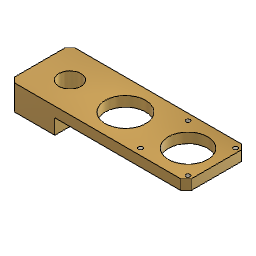
BC linear drive v5 (Autodesk Fusion 360 archive; units mm, degrees)
design "BC linear drive plate"
Autodesk Fusion 360 part; units mm, degrees
note: some values were not read from the file. Set by a fixed rule: the direction of a hole.
sketch "Sketch1" plane through (0, 0, 0) normal (0, 1, 0) x (1, 0, 0)
  circle A0 centre (0, 0) radius 20
  circle A1 centre (-55, 0) radius 16 construction
  circle A2 centre (-55, 0) radius 11
  line L0 (0, 0) -> (-55, 0) construction
  line L1 (-85, 30) -> (90, 30)
  line L2 (90, 30) -> (90, -30)
  line L3 (90, -30) -> (-85, -30)
  line L4 (-85, -30) -> (-85, 30)
  line L5 (-40, 30) -> (-40, -30)
  line L6 (-66.3137, -11.3137) -> (-43.6863, 11.3137) construction
  line L7 (-66.3137, 11.3137) -> (-43.6863, -11.3137) construction
  line L8 (-55, 16) -> (-55, -16) construction
  line L9 (38.43, -23.57) -> (85.57, -23.57) construction
  line L10 (85.57, -23.57) -> (85.57, 23.57) construction
  line L11 (85.57, 23.57) -> (38.43, 23.57) construction
  line L12 (38.43, 23.57) -> (38.43, -23.57) construction
  line L13 (38.43, 23.57) -> (85.57, -23.57) construction
  circle A3 centre (62, 0) radius 19.5
  point P0 (-66.3137, 11.3137)
  point P1 (-55, 16)
  point P2 (-43.6863, 11.3137)
  point P3 (-43.6863, -11.3137)
  point P4 (-55, -16)
  point P5 (-66.3137, -11.3137)
  dimension "d1" = 32
  dimension "d2" = 22
  dimension "d3" = 55
  dimension "d4" = 40
  dimension "d5" = 60
  dimension "d6" = 30
  dimension "d7" = 90
  dimension "d8" = 15
  dimension "d9" = 45
  dimension "d20" = 47.14
  dimension "d22" = 39
  dimension "d27" = 62
  constraint coincident A0.centre L0.start
  constraint concentric A1 A2
  constraint coincident A1.centre A2.centre
  constraint horizontal L0
  constraint horizontal L1
  constraint vertical L2
  constraint horizontal L3
  constraint vertical L4
  constraint symmetric L0 L1 L3
  constraint coincident L1 L5.start
  constraint coincident L3 L5.end
  constraint perpendicular L3 L5
  constraint coincident A1 P5
  constraint coincident A1 P2
  constraint coincident A1 P0
  constraint coincident A1 P3
  constraint coincident A1 P1
  constraint coincident A1 P4
  constraint coincident A1.centre L6
  constraint perpendicular L6 L7
  constraint coincident A1.centre L7
  constraint vertical L8
  constraint coincident A1.centre L8
  constraint coincident P0 L7.start
  constraint coincident P1 L8.start
  constraint coincident P2 L6.end
  constraint coincident P3 L7.end
  constraint coincident P4 L8.end
  constraint coincident P5 L6.start
  constraint horizontal L9
  constraint vertical L10
  constraint horizontal L11
  constraint vertical L12
  constraint equal L9 L12
  constraint symmetric L0 L9 L11
  constraint midpoint L13 A3.centre
  measures "d1" diameter of A1
  measures "d2" diameter of A2
  measures "d3" distance of A0.centre A1.centre
  measures "d4" diameter of A0
  measures "d5" distance of L1.start L3.end
  measures "d6" distance of A1.centre L4
  measures "d7" distance of A0.centre L2
  measures "d8" distance of A1.centre L5
  measures "d9" angle of L7 L8
  measures "d20" distance of L9.start L9.end
  measures "d22" diameter of A3
  measures "d27" distance of A0.centre A3.centre
extrude "Extrude1" add sketch "Sketch1" along normal blind 25
extrude "Extrude3" cut sketch "Sketch1" along normal blind 15 contours L1 L2 L3 L5 | A3
hole "Hole1" at (-66.3137, 0, 11.3137) at (-55, 0, 16) at (-66.3137, 0, -11.3137) at (-55, 0, -16) at (-43.6863, 0, -11.3137) at (-43.6863, 0, 11.3137) direction (0, 1, 0) diameter 3.332 depth 15 tip angle 118
thread "Thread1" "ISO Metric profile 4.0 M4x0.7 6H"
hole "Hole2" at (38.43, 0, 23.57) at (38.43, 0, -23.57) at (85.57, 0, 23.57) at (85.57, 0, -23.57) direction (0, 1, 0) diameter 4.234 depth 60 tip angle 118
thread "Thread2" "ISO Metric profile 5.0 M5x0.8 6H"
chamfer "Chamfer1" distance 5 angle 45 4 edges at (-85, 12.5, -30) (-85, 12.5, 30) (90, 20, -30) (90, 20, 30)

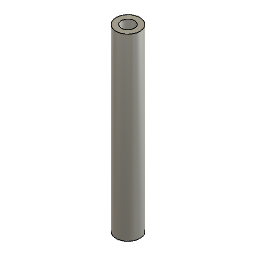
design "BC linaer drive motor spacer"
Autodesk Fusion 360 part; units mm, degrees
cylinder "CylinderPrimitive1" add diameter 10 height 75 placed x (1, 0, 0) y (0, 0, -1) z (0, 1, 0) at (0, 0, 0)
hole "Hole1" at (0, 0, 0) direction (0, 1, 0) diameter 5.5 end through all

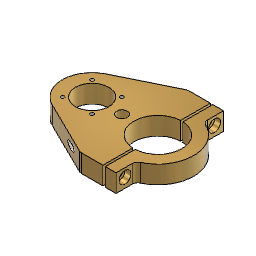
design "BC linear drive top bearing fixture"
Autodesk Fusion 360 part; units mm, degrees
sketch "Sketch1" plane through (0, 0, 0) normal (0, 1, 0) x (1, 0, 0)
  circle A0 centre (0, 0) radius 17.5 construction
  line L0 (-12.3744, 12.3744) -> (12.3744, 12.3744) construction
  line L1 (12.3744, 12.3744) -> (12.3744, -12.3744) construction
  line L2 (12.3744, -12.3744) -> (-12.3744, -12.3744) construction
  line L3 (-12.3744, -12.3744) -> (-12.3744, 12.3744) construction
  circle A1 centre (0, 0) radius 14
  circle A2 centre (55, 0) radius 20
  line L4 (65, 28.2843) -> (65, 45)
  line L5 (65, 45) -> (35, 45)
  line L6 (35, 45) -> (-11.0043, 22.4478)
  arc A3 (-11.0043, 22.4478) -> (-25, 0) centre (0, 0) ccw
  arc A4 (85, 0) -> (65, 28.2843) centre (55, 0) ccw
  line L7 (1.75, 0) -> (22.5, 0)
  arc A5 (65, -28.2843) -> (85, 0) centre (55, 0) ccw
  line L8 (65, -28.2843) -> (65, -45)
  line L9 (65, -45) -> (35, -45)
  line L10 (35, -45) -> (-11.0043, -22.4478)
  arc A6 (-25, 0) -> (-11.0043, -22.4478) centre (0, 0) ccw
  point P0 (25, 0)
  dimension "d1" = 35
  dimension "d2" = 28
  dimension "d3" = 40
  dimension "d4" = 55
  dimension "d5" = 25
  dimension "d6" = 30
  dimension "d7" = 10
  dimension "d8" = 30
  dimension "d9" = 45
  dimension "d31" = 30
  constraint coincident A0.centre A1.centre
  constraint horizontal L0
  constraint vertical L1
  constraint horizontal L2
  constraint vertical L3
  constraint coincident A0 L1.end
  constraint coincident A0 L0.start
  constraint equal L0 L1
  constraint coincident A0 L0.end
  constraint concentric A0 A1
  constraint horizontal A0.centre A2.centre
  constraint vertical L4
  constraint perpendicular L4 L5
  constraint tangent L6 A3
  constraint coincident A2.centre A4.centre
  constraint horizontal A2.centre A4.start
  constraint horizontal A0.centre A3.end
  constraint symmetric L4.start L7 A5.start
  constraint symmetric L4.end L7 L8.end
  constraint symmetric L5.end L7 L9.end
  constraint symmetric L6.end L7 L10.end
  constraint symmetric A3.end L7 A6.start
  constraint symmetric A3 L7 A6
  constraint symmetric A4.start L7 A5.end
  constraint symmetric A4 L7 A5
  constraint horizontal A2.centre P0
  measures "d1" diameter of A0
  measures "d2" diameter of A1
  measures "d3" diameter of A2
  measures "d4" distance of A0.centre A2.centre
  measures "d5" radius of A3
  measures "d6" radius of A4
  measures "d7" distance of A2.centre L4
  measures "d8" distance of L4.end L5.end
  measures "d9" distance of A2.centre L5
  measures "d31" distance of A2.centre P0
extrude "Extrude1" add sketch "Sketch1" along normal blind 15 makes body 1
hole "Hole1" at (-12.3744, 0, 12.3744) at (12.3744, 0, 12.3744) at (12.3744, 0, -12.3744) at (-12.3744, 0, -12.3744) direction (0, 1, 0) diameter 2.93 end through all bodies 1
thread "Thread2" "ISO Metric profile 3.5 M3.5x0.6 6H"
ref_plane "WorkPlane1" through (55, 0, 0) normal (1, 0, 0) x (0, 1, 0)
sketch "Sketch2" plane through (55, 0, 0) normal (1, 0, 0) x (0, 0, -1)
  line L0 (-52.531, 37.047) -> (45, 37.047)
  line L1 (45, 37.047) -> (45, -15)
  line L2 (45, -15) -> (-52.531, -15)
  line L3 (-52.531, -15) -> (-52.531, 37.047)
  constraint horizontal L0
  constraint vertical L1
  constraint horizontal L2
  constraint vertical L3
extrude "Extrude2" cut sketch "Sketch2" along normal mid plane 2 bodies 1 makes body 2 at (73.8112, 10, -23.3696)
sketch "Sketch3" plane through (65, 0, 0) normal (1, 0, 0) x (0, 0, -1)
  line L0 (28.2843, 0) -> (45, 0)
  line L1 (45, 0) -> (45, 15)
  line L2 (45, 15) -> (28.2843, 15)
  line L3 (28.2843, 15) -> (28.2843, 0)
  point P0 (37.5, 8)
  dimension "d23" = 7.5
  measures "d23" distance of L1 P0
hole "Hole2" at (65, 8, -37.5) direction (-1, 0, 0) diameter 5.5 depth 10 tip angle 180 counterbore diameter 10 counterbore depth 5 bodies 2
hole "Hole3" at (65, 8, -37.5) direction (-1, 0, 0) diameter 5.029 end through all bodies 1
thread "Thread1" "ISO Metric profile 5.5 M5.5x0.5 6H"
mirror "Mirror1" about plane through (0, 0, 0) normal (0, 0, 1) of "Hole2", "Hole3"
fillet "Fillet1" radius 5 4 edges at (35, 7.5, -45) (35, 7.5, 45) (65, 7.5, -28.2843) (65, 7.5, 28.2843) on bodies 1 2
hole "Hole4" at (25, 0, 0) direction (0, 1, 0) diameter 9 end through all bodies 1
copy_body "Body->Comp1" bodies 1 removing the originals makes body 3 in component "console"
copy_body "Body->Comp2" bodies 2 removing the originals makes body 4 in component "brace"
component "console" placed x (1, 0, 0) y (0, 1, 0) z (0, 0, 1) at (0, 0, 0)
component "brace" placed x (1, 0, 0) y (0, 1, 0) z (0, 0, 1) at (0, 0, 0)
named bodies: "console", "brace"

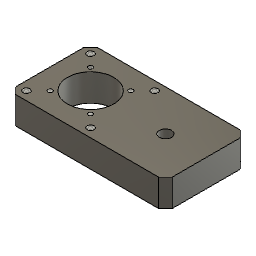
design "BC linear drive bottom bracket"
Autodesk Fusion 360 part; units mm, degrees
sketch "Sketch1" plane through (0, 0, 0) normal (0, 1, 0) x (1, 0, 0)
  circle A0 centre (-55, 0) radius 17
  line L0 (-78.57, 23.57) -> (-31.43, 23.57) construction
  line L1 (-31.43, 23.57) -> (-31.43, -23.57) construction
  line L2 (-31.43, -23.57) -> (-78.57, -23.57) construction
  line L3 (-78.57, -23.57) -> (-78.57, 23.57) construction
  line L4 (-78.57, -23.57) -> (-31.43, 23.57) construction
  line L5 (-85, 30) -> (30, 30)
  line L6 (30, 30) -> (30, -30)
  line L7 (30, -30) -> (-85, -30)
  line L8 (-85, -30) -> (-85, 30)
  line L9 (0, 0) -> (-55, 0) construction
  circle A1 centre (-55, 0) radius 21 construction
  line L10 (-78.57, 23.57) -> (-31.43, -23.57) construction
  line L11 (-55, 23.57) -> (-55, -23.57) construction
  line L12 (-78.57, 0) -> (-31.43, 0) construction
  point P0 (-55, 21)
  point P1 (-69.8492, 14.8492)
  point P2 (-76, 0)
  point P3 (-69.8492, -14.8492)
  point P4 (-55, -21)
  point P5 (-40.1508, -14.8492)
  point P6 (-40.1508, 14.8492)
  point P7 (-34, 0)
  dimension "d2" = 34
  dimension "d3" = 55
  dimension "d4" = 47.14
  dimension "d5" = 30
  dimension "d6" = 30
  dimension "d7" = 60
  dimension "d20" = 42
  constraint horizontal L0
  constraint vertical L1
  constraint horizontal L2
  constraint vertical L3
  constraint equal L2 L3
  constraint midpoint A0.centre L4
  constraint horizontal L5
  constraint vertical L6
  constraint horizontal L7
  constraint vertical L8
  constraint coincident L9.start origin
  constraint coincident A0.centre L9.end
  constraint symmetric L5 L7 L9
  constraint midpoint L0 L11.start
  constraint midpoint L2 L11.end
  constraint midpoint L3 L12.start
  constraint midpoint L1 L12.end
  constraint coincident A1 P0
  constraint coincident L11 P0
  constraint coincident A1 P1
  constraint coincident L10 P1
  constraint coincident A1 P2
  constraint coincident L12 P2
  constraint coincident A1 P3
  constraint coincident L4 P3
  constraint coincident L11 P4
  constraint coincident A1 P4
  constraint coincident A1 P5
  constraint coincident L10 P5
  constraint coincident A1 P6
  constraint coincident L4 P6
  constraint coincident A1 P7
  constraint coincident L9 P7
  measures "d2" diameter of A0
  measures "d3" distance of L9.start A0.centre
  measures "d4" distance of L1.end L2.end
  measures "d5" distance of L9.start L6
  measures "d6" distance of A0.centre L8
  measures "d7" distance of L5.end L6.end
  measures "d20" diameter of A1
extrude "Extrude1" add sketch "Sketch1" along normal blind 20
hole "Hole1" at (0, 0, 0) direction (0, 1, 0) diameter 9 end through all
hole "Hole2" at (-31.43, 0, 23.57) at (-31.43, 0, -23.57) at (-78.57, 0, -23.57) at (-78.57, 0, 23.57) direction (0, 1, 0) diameter 5.029 end through all
thread "Thread3" "ISO Metric profile 5.5 M5.5x0.5 6H"
hole "Hole3" at (-69.8492, 0, 14.8492) at (-69.8492, 0, -14.8492) at (-40.1508, 0, -14.8492) at (-40.1508, 0, 14.8492) direction (0, 1, 0) diameter 3.332 end through all
thread "Thread2" "ISO Metric profile 4.0 M4x0.7 6H"
chamfer "Chamfer3" distance 5 angle 45 4 edges at (-85, 10, 30) (-85, 10, -30) (30, 10, 30) (30, 10, -30)
